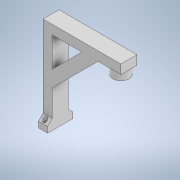
# Autodesk Inventor part: main_stand_upper_half
Saved by Autodesk Inventor 2021 (Build 250183000, 183)
## iProperties
Created: 2020-10-10
Part Number: main_stand_upper_half
Material: Generic
Document SubType Name: Modeling
Designer: bober
Density: 1 g/cm^3
Appearance: Default
Author: bober
Autodesk Inventor part; units mm, degrees
ref_plane "YZ Plane" through (0, 0, 0) normal (1, 0, 0) x (0, 1, 0)
ref_plane "XZ Plane" through (0, 0, 0) normal (0, 1, 0) x (-1, 0, 0)
ref_plane "XY Plane" through (0, 0, 0) normal (0, 0, 1) x (1, 0, 0)
sketch "Sketch1" plane through (0, 0, 0) normal (0, 1, 0) x (-1, 0, 0)
  line L0 (-10, 27.5) -> (10, 27.5)
  line L1 (10, 27.5) -> (10, -27.5)
  line L2 (10, -27.5) -> (-10, -27.5)
  line L3 (-10, -27.5) -> (-10, 27.5)
  line L4 (-10, 27.5) -> (10, -27.5) construction
  line L5 (10, 27.5) -> (-10, -27.5) construction
  point P0 (0, 0)
  dimension "d0" = 20
  dimension "d1" = 55
  constraints: 12 end point, 2 midpoint, 2 parallel, 1 horizontal, 1 perpendicular
  measures "d0" distance of L1.end L2.end
  measures "d1" distance of L0.end L1.end
extrude "Extrusion1" add sketch "Sketch1" along normal blind 3
sketch "Sketch2" plane through (0, 3, 0) normal (0, 1, 0) x (1, 0, 0)
  circle A0 centre (0, -22.5) radius 2
  circle A1 centre (0, 22.5) radius 2
  point P0 (0, 0)
  dimension "d4" = 4
  dimension "d5" = 4
  constraints: 2 centre point
  measures "d4" diameter of A0
  measures "d5" diameter of A1
extrude "Extrusion2" cut sketch "Sketch2" against normal blind 3
sketch "Sketch3" plane through (0, 3, 0) normal (0, 1, 0) x (1, 0, 0)
  line L0 (10, -17.5) -> (-10, -17.5)
  line L1 (-10, -17.5) -> (-10, 17.5)
  line L2 (-10, 17.5) -> (10, 17.5)
  line L3 (10, 17.5) -> (10, -17.5)
  line L4 (10, -17.5) -> (-10, 17.5) construction
  line L5 (-10, -17.5) -> (10, 17.5) construction
  point P0 (0, 0)
  dimension "d8" = 20
  dimension "d9" = 35
  constraints: 12 end point, 2 midpoint, 2 parallel, 1 horizontal, 1 perpendicular
  measures "d8" distance of L1.end L2.end
  measures "d9" distance of L0.end L1.end
extrude "Extrusion3" add sketch "Sketch3" along normal blind 178
sketch "Sketch4" plane through (0, 181, 0) normal (0, 1, 0) x (1, 0, 0)
  line L0 (-10, 17.5) -> (-10, -17.5) projected
  line L1 (-10, -17.5) -> (160, -17.5)
  line L2 (160, -17.5) -> (160, 17.5)
  line L3 (160, 17.5) -> (-10, 17.5)
  line L4 (-10, 17.5) -> (-10, -17.5)
  point P0 (0, 0)
  dimension "d12" = 170
  dimension "d13" = 35
  constraints: 8 end point, 2 parallel, 1 horizontal, 1 perpendicular
  measures "d12" distance of L3.end L2.end
  measures "d13" distance of L2.end L1.end
extrude "Extrusion4" add sketch "Sketch4" along normal blind 10
sketch "Sketch5" plane through (0, 181, 0) normal (0, -1, 0) x (1, 0, 0)
  circle A0 centre (142.5, 0) radius 17.5
  point P0 (0, 0)
  constraints: 1 centre point
extrude "Extrusion5" add sketch "Sketch5" along normal blind 17
thicken "Thicken1" operation add thickness 10 both sides no extend neighbours yes toward (0, 1, 0) faces at (46.6667, 191, -5.8333)
thicken "Thicken2" operation add thickness 10 both sides no extend neighbours yes toward (0, 1, 0) faces at (7.3333, 3, 22.5) (7.3333, 3, -22.5)
sketch "Sketch8" plane through (0, 181, 0) normal (0, -1, 0) x (1, 0, 0)
  line L0 (75, 17.5) -> (110, 17.5)
  line L1 (110, 17.5) -> (110, -17.5)
  line L2 (110, -17.5) -> (75, -17.5)
  line L3 (75, -17.5) -> (75, 17.5)
  point P0 (0, 0)
  dimension "d34" = 35
  dimension "d35" = 35
  constraints: 8 end point, 2 parallel, 1 horizontal, 1 perpendicular
  measures "d34" distance of L1.end L2.end
  measures "d35" distance of L0.end L1.end
sketch "Sketch9" plane through (10, 0, 27.5) normal (1, 0, 0) x (0, 0, -1)
  line L0 (10, 116) -> (45, 116)
  line L1 (45, 116) -> (45, 81)
  line L2 (45, 81) -> (10, 81)
  line L3 (10, 81) -> (10, 116)
  point P0 (27.5, 0)
  dimension "d36" = 35
  dimension "d37" = 35
  constraints: 8 end point, 2 parallel, 1 horizontal, 1 perpendicular
  measures "d36" distance of L1.end L2.end
  measures "d37" distance of L0.end L1.end
loft "Loft3" add profiles "Sketch9", "Sketch8"
sketch "Sketch10" plane through (-10, 13, 17.5) normal (0, 1, 0) x (1, 0, 0)
  line L0 (20, 0) -> (20, 35) projected
  line L1 (0, 0) -> (0, -10) projected
  line L2 (20, 0) -> (0, 0)
  line L3 (0, 0) -> (0, -10)
  line L4 (0, -10) -> (20, -10)
  line L5 (20, -10) -> (20, 0)
  line L6 (20, -10) -> (20, 45) projected
  line L7 (170, 35) -> (0, 35) projected
  line L8 (20, 45) -> (0, 45)
  line L9 (0, 45) -> (0, 35)
  line L10 (0, 35) -> (20, 35)
  line L11 (20, 35) -> (20, 45)
  point P0 (10, 17.5)
  constraints: 16 end point, 4 parallel, 2 horizontal, 2 perpendicular
extrude "Extrusion6" add sketch "Sketch10" along normal blind 10
chamfer "Chamfer1" distance 10 angle 45 2 edges at (0, 23, -27.5) (0, 23, 27.5)
sketch "Sketch11" plane through (0, 13, -22.5) normal (0, -1, 0) x (1, 0, 0)
  circle A0 centre (0, 0) radius 2 projected
  circle A1 centre (0, 0) radius 4
  circle A2 centre (0, 45) radius 2 projected
  circle A3 centre (0, 45) radius 4
  point P0 (0, 22.5)
  dimension "d47" = 8
  dimension "d48" = 8
  constraints: 2 centre point, 2 coincident
  measures "d47" diameter of A1
  measures "d48" diameter of A3
extrude "Extrusion7" cut sketch "Sketch11" against normal blind 10 contours A0 | A1 | A2 | A3
body "Solid1"
